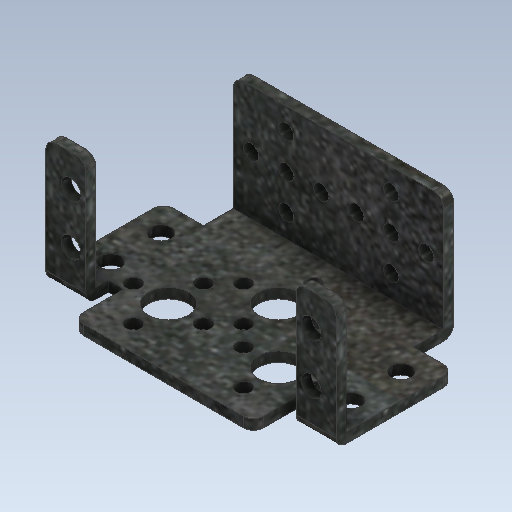
# Autodesk Inventor part: Деталь4
Saved by Autodesk Inventor 2020.1 (Build 241239000, 239)
## iProperties
Created: 2021-08-12
Part Number: Деталь4
Material: Сталь
Document SubType Name: Modeling
Designer: User
Density: 7.85 g/cm^3
Appearance: Листовая
Author: User
Autodesk Inventor part; units mm, degrees
ref_plane "YZ Plane" through (0, 0, 0) normal (1, 0, 0) x (0, 1, 0)
ref_plane "XZ Plane" through (0, 0, 0) normal (0, 1, 0) x (-1, 0, 0)
ref_plane "XY Plane" through (0, 0, 0) normal (0, 0, 1) x (1, 0, 0)
sketch "Эскиз2" plane through (0, 0, 0) normal (0, 1, 0) x (-1, 0, 0)
  line L0 (0, 0) -> (-58, 0)
  line L1 (-58, 0) -> (-58, 37)
  line L2 (-58, 37) -> (0, 37)
  line L3 (0, 37) -> (0, 0)
  line L4 (-58, 8) -> (-50, 8)
  line L5 (-50, 8) -> (-50, 0)
  line L6 (-50, 0) -> (-58, 0)
  line L7 (-58, 0) -> (-58, 8)
  line L8 (-58, 37) -> (-47, 37)
  line L9 (-47, 37) -> (-47, 27)
  line L10 (-47, 27) -> (-58, 27)
  line L11 (-58, 27) -> (-58, 37)
  line L12 (-50, 27) -> (-58, 27)
  line L13 (-58, 27) -> (-58, 31.5)
  line L14 (-58, 31.5) -> (-50, 31.5)
  line L15 (-50, 31.5) -> (-50, 27)
  line L16 (0, 37) -> (-11, 37)
  line L17 (-11, 37) -> (-11, 27)
  line L18 (-11, 27) -> (0, 27)
  line L19 (0, 27) -> (0, 37)
  line L20 (-11, 27) -> (-7.6324, 27)
  line L21 (-11, 31.5) -> (-11, 27)
  line L22 (0, 27) -> (-8, 27)
  line L23 (-8, 27) -> (-8, 31.5)
  line L24 (-8, 31.5) -> (0, 31.5)
  line L25 (0, 31.5) -> (0, 27)
  line L26 (-8, 8) -> (0, 8)
  line L27 (0, 8) -> (0, 0)
  line L28 (0, 0) -> (-8, 0)
  line L29 (-8, 0) -> (-8, 8)
  point P0 (0, 31.5)
  dimension "d0" = 58
  dimension "d1" = 37
  dimension "d2" = 8
  dimension "d3" = 8
  dimension "d4" = 10
  dimension "d5" = 11
  dimension "d6" = 4.5
  dimension "d7" = 10
  dimension "d8" = 11
  dimension "d9" = 8
  constraints: 60 end point, 14 parallel, 8 horizontal, 7 perpendicular, 4 point on line
  measures "d0" distance of L0.start L0.end
  measures "d1" distance of L2.end L0.start
  measures "d2" distance of L4.start L4.end
  measures "d3" distance of L4.end L5.end
  measures "d4" distance of L8.end L9.end
  measures "d5" distance of L9.end L10.end
  measures "d6" distance of L14.end L12.start
  measures "d7" distance of L16.end L17.end
  measures "d8" distance of L17.end L18.end
  measures "d9" distance of L23.end L24.end
extrude "Выдавливание1" add sketch "Эскиз2" along normal blind 2 contours L0 L5 L4 L1 L10 L9 L2 L17 L18 L3 L26 L29 | L18 L23 L24 L3 | L1 L14 L15 L10
sketch "Эскиз3" plane through (0, 2, 0) normal (0, 1, 0) x (1, 0, 0)
  line L0 (0, -31.5) -> (8, -31.5) projected
  line L1 (0, -8) -> (0, -31.5) projected
  line L2 (8, -31.5) -> (0, -31.5)
  line L3 (0, -31.5) -> (0, -29.5)
  line L4 (0, -29.5) -> (8, -29.5)
  line L5 (8, -29.5) -> (8, -31.5)
  line L6 (50, -31.5) -> (58, -31.5) projected
  line L7 (58, -31.5) -> (58, -8) projected
  line L8 (50, -31.5) -> (58, -31.5)
  line L9 (58, -31.5) -> (58, -29.5)
  line L10 (58, -29.5) -> (50, -29.5)
  line L11 (50, -29.5) -> (50, -31.5)
  line L12 (50, 0) -> (8, 0) projected
  line L13 (8, 0) -> (8, -8) projected
  line L14 (50, 0) -> (8, 0)
  line L15 (8, 0) -> (8, -2)
  line L16 (8, -2) -> (50, -2)
  line L17 (50, -2) -> (50, 0)
  point P0 (0, 0)
  dimension "d12" = 2
  dimension "d13" = 2
  constraints: 24 end point, 6 parallel, 3 horizontal, 3 perpendicular, 3 point on line
  measures "d12" distance of L0.end L4.end
  measures "d13" distance from line of L12 L15.end
extrude "Выдавливание2" add sketch "Эскиз3" along normal blind 23
sketch "Эскиз4" plane through (50, 0, 31.5) normal (0, 0, 1) x (1, 0, 0)
  line L0 (-42, 2) -> (-50, 2) projected
  line L1 (-42, 0) -> (-42, 25) projected
  line L2 (-42, 2) -> (-42, 25)
  line L3 (0, 0) -> (0, 25) projected
  circle A0 centre (-45, 18.5) radius 2
  circle A1 centre (-45, 8.5) radius 2
  circle A2 centre (3, 18.5) radius 2
  circle A3 centre (3, 8.5) radius 2
  point P0 (-50, 0)
  point P1 (-42, 13.5)
  point P2 (0, 13.5)
  dimension "d16" = 4
  dimension "d17" = 5
  dimension "d18" = 3
  dimension "d19" = 4
  dimension "d20" = 5
  dimension "d21" = 4
  dimension "d22" = 5
  dimension "d23" = 3
  dimension "d24" = 4
  constraints: 4 centre point, 2 end point, 1 collinear, 1 midpoint, 1 point on line
  measures "d16" diameter of A0
  measures "d17" vertical distance of A0.centre point (-42, 13.5)
  measures "d18" horizontal distance of A0.centre point (-42, 13.5)
  measures "d19" diameter of A1
  measures "d20" vertical distance of point (-42, 13.5) A1.centre
  measures "d21" diameter of A2
  measures "d22" vertical distance of A2.centre point (0, 13.5)
  measures "d23" distance from line of L3 A2.centre
  measures "d24" diameter of A3
extrude "Выдавливание3" cut sketch "Эскиз4" against normal blind 10
sketch "Эскиз6" plane through (50, 0, 0) normal (0, 0, -1) x (-1, 0, 0)
  line L0 (0, 2) -> (0, 25) projected
  line L1 (42, 25) -> (0, 25) projected
  circle A0 centre (24.5, 13.5) radius 1.5
  circle A1 centre (17.5, 13.5) radius 1.5
  circle A2 centre (31.5, 13.5) radius 1.5
  circle A3 centre (38.5, 13.5) radius 1.5
  circle A4 centre (10.5, 13.5) radius 1.5
  circle A5 centre (3.5, 13.5) radius 1.5
  circle A6 centre (10.5, 20.5) radius 1.5
  circle A7 centre (10.5, 6.5) radius 1.5
  circle A8 centre (31.5, 20.5) radius 1.5
  circle A9 centre (31.5, 6.5) radius 1.5
  point P0 (50, 0)
  point P1 (0, 13.5)
  point P2 (21, 25)
  point P3 (21, 13.5)
  dimension "d27" = 3
  dimension "d28" = 3
  dimension "d29" = 3.5
  dimension "d30" = 3.5
  dimension "d31" = 3
  dimension "d32" = 3
  dimension "d33" = 3
  dimension "d34" = 3
  dimension "d35" = 7
  dimension "d36" = 7
  dimension "d37" = 7
  dimension "d38" = 0
  dimension "d39" = 7
  dimension "d40" = 3
  dimension "d41" = 3
  dimension "d42" = 7
  dimension "d43" = 7
  dimension "d44" = 3
  dimension "d45" = 3
  constraints: 10 centre point, 2 midpoint
  measures "d27" diameter of A0
  measures "d28" diameter of A1
  measures "d29" distance of A0.centre point (21, 13.5)
  measures "d30" distance of A1.centre point (21, 13.5)
  measures "d31" diameter of A2
  measures "d32" diameter of A3
  measures "d33" diameter of A4
  measures "d34" diameter of A5
  measures "d35" distance of A2.centre A0.centre
  measures "d36" distance of A3.centre A2.centre
  measures "d37" distance of A4.centre A1.centre
  measures "d38" horizontal distance of point (21, 25) point (21, 13.5)
  measures "d39" distance of A5.centre A4.centre
  measures "d40" diameter of A6
  measures "d41" diameter of A7
  measures "d42" distance of A7.centre A4.centre
  measures "d43" distance of A6.centre A4.centre
  measures "d44" diameter of A8
  measures "d45" diameter of A9
extrude "Выдавливание4" cut sketch "Эскиз6" against normal blind 10
sketch "Эскиз7" plane through (0, 2, 0) normal (0, 1, 0) x (1, 0, 0)
  circle A0 centre (5, -13.5) radius 2
  line L0 (8, -2) -> (8, -8) projected
  line L1 (8, -8) -> (0, -8) projected
  circle A1 centre (5, -23.5) radius 2
  circle A2 centre (53, -13.5) radius 2
  line L2 (50, -8) -> (50, -2) projected
  circle A3 centre (53, -23.5) radius 2
  line L3 (8, -2) -> (50, -2) projected
  circle A4 centre (29, -14) radius 4
  line L4 (11, -37) -> (47, -37) projected
  circle A5 centre (40, -25) radius 4
  line L5 (58, -29.5) -> (58, -8) projected
  circle A6 centre (18, -25) radius 4
  line L6 (0, -8) -> (0, -29.5) projected
  circle A7 centre (25, -25) radius 1.5
  circle A8 centre (33, -25) radius 1.5
  circle A9 centre (40, -32) radius 1.5
  circle A10 centre (47, -25) radius 1.5
  circle A11 centre (11, -25) radius 1.5
  circle A12 centre (18, -18) radius 1.5
  circle A13 centre (40, -18) radius 1.5
  circle A14 centre (18, -32) radius 1.5
  circle A15 centre (29, -21) radius 1.5
  circle A16 centre (36, -14) radius 1.5
  circle A17 centre (22, -14) radius 1.5
  circle A18 centre (29, -7) radius 1.5
  point P0 (0, 0)
  point P1 (29, -2)
  dimension "d48" = 4
  dimension "d49" = 3
  dimension "d50" = 5.5
  dimension "d51" = 4
  dimension "d52" = 10
  dimension "d53" = 4
  dimension "d54" = 3
  dimension "d55" = 4
  dimension "d56" = 8
  dimension "d57" = 23
  dimension "d58" = 8
  dimension "d59" = 12
  dimension "d60" = 18
  dimension "d61" = 8
  dimension "d62" = 18
  dimension "d63" = 3
  dimension "d64" = 3
  dimension "d65" = 3
  dimension "d66" = 3
  dimension "d67" = 3
  dimension "d68" = 3
  dimension "d69" = 7
  dimension "d70" = 7
  dimension "d71" = 7
  dimension "d72" = 7
  dimension "d73" = 7
  dimension "d74" = 7
  dimension "d75" = 3
  dimension "d76" = 3
  dimension "d77" = 3
  dimension "d78" = 3
  dimension "d79" = 3
  dimension "d80" = 3
  dimension "d81" = 7
  dimension "d82" = 7
  dimension "d83" = 7
  dimension "d84" = 7
  constraints: 19 centre point, 1 midpoint
  measures "d48" diameter of A0
  measures "d49" distance from line of L0 A0.centre
  measures "d50" distance from line of L1 A0.centre
  measures "d51" diameter of A1
  measures "d52" distance of A0.centre A1.centre
  measures "d53" diameter of A2
  measures "d54" distance from line of L2 A2.centre
  measures "d55" diameter of A3
  measures "d56" diameter of A4
  measures "d57" distance from line of L4 A4.centre
  measures "d58" diameter of A5
  measures "d59" distance from line of L4 A5.centre
  measures "d60" distance from line of L5 A5.centre
  measures "d61" diameter of A6
  measures "d62" distance from line of L6 A6.centre
  measures "d63" diameter of A7
  measures "d64" diameter of A8
  measures "d65" diameter of A9
  measures "d66" diameter of A10
  measures "d67" diameter of A11
  measures "d68" diameter of A12
  measures "d69" distance of A12.centre A6.centre
  measures "d70" distance of A11.centre A6.centre
  measures "d71" distance of A7.centre A6.centre
  measures "d72" distance of A8.centre A5.centre
  measures "d73" distance of A9.centre A5.centre
  measures "d74" distance of A10.centre A5.centre
  measures "d75" diameter of A13
  measures "d76" diameter of A14
  measures "d77" diameter of A15
  measures "d78" diameter of A16
  measures "d79" diameter of A17
  measures "d80" diameter of A18
  measures "d81" distance of A15.centre A4.centre
  measures "d82" distance of A16.centre A4.centre
  measures "d83" distance of A4.centre A18.centre
  measures "d84" distance of A17.centre A4.centre
extrude "Выдавливание5" cut sketch "Эскиз7" against normal blind 10
fillet "Сопряжение1" radius 2 13 edges at (58, 25, 30.5) (50, 25, 30.5) (50, 25, 1) (8, 25, 1) (8, 25, 30.5) (0, 25, 30.5) (54, 0, 31.5) (4, 0, 31.5) (29, 0, 0) (58, 1, 8) (0, 1, 8) (11, 1, 37) (47, 1, 37)
